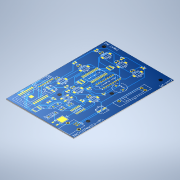
# Autodesk Inventor part: Buttom Case
Saved by Autodesk Inventor 2020 (Build 240168000, 168)
## iProperties
Created: 2019-11-08
Part Number: Buttom Case
Material: Generic
Document SubType Name: Modeling
Designer: siwat
Density: 1 g/cm^3
Appearance: Default
Author: siwat
Autodesk Inventor part; units mm, degrees
ref_plane "YZ Plane" through (0, 0, 0) normal (1, 0, 0) x (0, 1, 0)
ref_plane "XZ Plane" through (0, 0, 0) normal (0, 1, 0) x (-1, 0, 0)
ref_plane "XY Plane" through (0, 0, 0) normal (0, 0, 1) x (1, 0, 0)
sketch "Sketch1" plane through (0, 0, 0) normal (0, 1, 0) x (-1, 0, 0)
  line L0 (18.1492, 45.8732) -> (-56.6508, 45.8732)
  line L1 (-56.6508, 45.8732) -> (-56.6508, -64.2368)
  line L2 (-56.6508, -64.2368) -> (18.1492, -64.2368)
  line L3 (18.1492, -64.2368) -> (18.1492, 45.8732)
  point P0 (0, 0)
  dimension "d0" = 110.11
  dimension "d1" = 74.8
  constraints: 8 end point, 2 parallel, 1 horizontal, 1 perpendicular
  measures "d0" distance of L2.end L0.start
  measures "d1" distance of L0.start L0.end
extrude "Extrusion1" add sketch "Sketch1" along normal blind 1
sketch "Sketch2" plane through (0, 1, 0) normal (0, 1, 0) x (1, 0, 0)
  line L0 (-18.1492, -45.8732) -> (-18.1492, 64.2368) construction
  line L1 (-18.1492, 64.2368) -> (56.633, 64.2368) construction
  line L2 (56.633, 64.2368) -> (56.633, -45.8732) construction
  line L3 (56.633, -45.8732) -> (-18.1492, -45.8732) construction
  point P0 (0, 0)
  dimension "d6" = 110.11
  constraints: 1 coincident, 2 other
  measures "d6" distance of L0.start L0.end
decal "Decal1"
sketch "Sketch3" plane through (0, 0, 0) normal (0, -1, 0) x (1, 0, 0)
  point P0 (0, 0)
body "Solid1"
